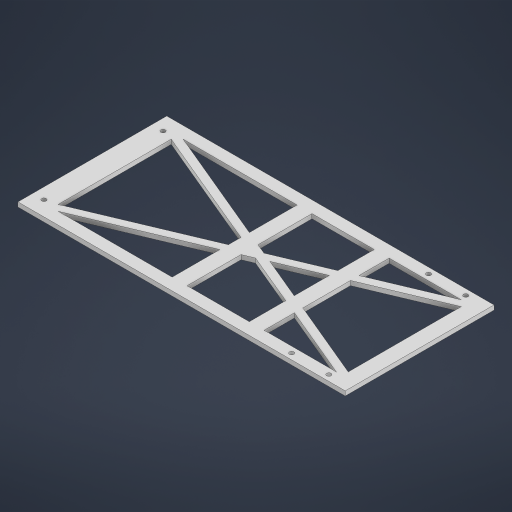
# Autodesk Inventor part: lf-esp
Saved by Autodesk Inventor 2023 (Build 270158000, 158)
## iProperties
Created: 2023-11-15
Part Number: lf-esp
Material: Ogólny
Document SubType Name: Modeling
Designer: mt150
Density: 1 g/cm^3
Appearance: Domyślna
Author: mt150
Autodesk Inventor part; units mm, degrees
ref_plane "YZ Plane" through (0, 0, 0) normal (1, 0, 0) x (0, 1, 0)
ref_plane "XZ Plane" through (0, 0, 0) normal (0, 1, 0) x (-1, 0, 0)
ref_plane "XY Plane" through (0, 0, 0) normal (0, 0, 1) x (1, 0, 0)
sketch "Szkic1" plane through (0, 0, 0) normal (0, 1, 0) x (-1, 0, 0)
  point P0 (0, 0)
sketch "Szkic2" plane through (0, 0, 0) normal (0, 1, 0) x (-1, 0, 0)
  line L0 (0, 0) -> (-15, 0)
  line L1 (-15, 0) -> (-15, 100)
  line L2 (-15, 100) -> (0, 100)
  line L3 (0, 100) -> (0, 0)
  line L4 (-7.5, 100) -> (-7.5, 90) construction
  line L5 (-7.5, 0) -> (-7.5, 10) construction
  circle A0 centre (-7.5, 90) radius 1.5
  circle A1 centre (-7.5, 10) radius 1.5
  line L6 (-15, 100) -> (-220, 100)
  line L7 (-220, 100) -> (-220, 92)
  line L8 (-220, 92) -> (-15, 92)
  line L9 (-15, 92) -> (-15, 100)
  line L10 (-15, 0) -> (-220, 0)
  line L11 (-220, 0) -> (-220, 8)
  line L12 (-220, 8) -> (-15, 8)
  line L13 (-15, 8) -> (-15, 0)
  line L14 (-15, 92) -> (-19, 92) construction
  line L15 (-15, 92) -> (-15, 88) construction
  line L16 (-220, 8) -> (-216, 8) construction
  line L17 (-220, 8) -> (-210, 8)
  line L18 (-210, 8) -> (-210, 92)
  line L19 (-210, 92) -> (-220, 92)
  line L20 (-220, 92) -> (-220, 8)
  line L21 (-210, 8) -> (-206, 8) construction
  line L22 (-210, 8) -> (-210, 12) construction
  line L23 (-15, 88) -> (-206, 8)
  line L24 (-19, 92) -> (-210, 12)
  line L25 (-15, 8) -> (-15, 12) construction
  line L26 (-15, 8) -> (-19, 8) construction
  line L27 (-210, 92) -> (-206, 92) construction
  line L28 (-210, 92) -> (-210, 88) construction
  line L29 (-210, 88) -> (-19, 8)
  line L30 (-15, 12) -> (-206, 92)
  line L31 (-220, 96) -> (-205, 96) construction
  line L32 (-220, 4) -> (-205, 4) construction
  circle A2 centre (-205, 96) radius 1.5
  circle A3 centre (-205, 4) radius 1.5
  line L33 (-205, 96) -> (-180, 96) construction
  line L34 (-205, 4) -> (-180, 4) construction
  circle A4 centre (-180, 96) radius 1.5
  circle A5 centre (-180, 4) radius 1.5
  line L35 (-220, 100) -> (-95, 100) construction
  line L36 (-95.6423, 92) -> (-105.6423, 92)
  line L37 (-105.6423, 92) -> (-105.6423, 8)
  line L38 (-105.6423, 8) -> (-95.6423, 8)
  line L39 (-95.6423, 8) -> (-95.6423, 92)
  line L40 (-220, 0) -> (-157.5, 0) construction
  line L41 (-157.5, 8) -> (-147.5, 8)
  line L42 (-147.5, 8) -> (-147.5, 92)
  line L43 (-147.5, 92) -> (-157.5, 92)
  line L44 (-157.5, 92) -> (-157.5, 8)
  point P0 (-105.725, 50)
  point P1 (-105.6423, 50.0346)
  point P2 (-105.6423, 49.9654)
  point P3 (-112.5, 52.8377)
  point P4 (-147.5, 67.4974)
  point P5 (-105.6423, 55.71)
  point P6 (-119.275, 50)
  point P7 (-147.5, 38.178)
  point P8 (-147.5, 61.822)
  point P9 (-112.5, 47.1623)
  point P10 (-105.6423, 44.29)
  point P11 (-147.5, 32.5026)
  point P12 (-157.5, 66.0105)
  point P13 (-157.5, 33.9895)
  point P14 (-157.5, 28.3141)
  point P15 (-157.5, 71.6859)
  point P16 (-95.6423, 59.8985)
  point P17 (-95.6423, 45.7769)
  point P18 (-95.6423, 54.2231)
  point P19 (-95.6423, 40.1015)
  dimension "d0" = 15
  dimension "d1" = 100
  dimension "d2" = 10
  dimension "d3" = 10
  dimension "d4" = 3
  dimension "d5" = 3
  dimension "d6" = 205
  dimension "d7" = 8
  dimension "d8" = 205
  dimension "d9" = 8
  dimension "d10" = 4
  dimension "d11" = 4
  dimension "d12" = 4
  dimension "d13" = 10
  dimension "d14" = 4
  dimension "d15" = 4
  dimension "d16" = 4
  dimension "d17" = 4
  dimension "d18" = 207.0773
  dimension "d19" = 15
  dimension "d20" = 15
  dimension "d21" = 3
  dimension "d22" = 3
  dimension "d23" = 25
  dimension "d24" = 3
  dimension "d25" = 3
  dimension "d26" = 125
  dimension "d27" = 10
  dimension "d28" = 10
  constraints: 90 end point, 16 point on line, 13 parallel, 10 horizontal, 6 centre point, 6 coincident, 6 perpendicular, 4 midpoint, 2 vertical
  measures "d0" distance of L1.end L2.end
  measures "d1" distance of L0.end L1.end
  measures "d2" distance of L4.start L4.end
  measures "d3" distance of L5.start L5.end
  measures "d4" diameter of A0
  measures "d5" diameter of A1
  measures "d6" distance of L8.end L7.end
  measures "d7" distance of L6.end L7.end
  measures "d8" distance of L11.end L12.end
  measures "d9" distance of L10.end L11.end
  measures "d10" distance of L8.end L14.end
  measures "d11" distance of L8.end L15.end
  measures "d12" distance of L11.end L16.end
  measures "d13" distance of L19.end L18.end
  measures "d14" distance of L17.end L21.end
  measures "d15" distance of L17.end L22.end
  measures "d16" distance of L12.end L25.end
  measures "d17" distance of L12.end L26.end
  measures "d18" distance of L25.end L27.end
  measures "d19" distance of L31.start L31.end
  measures "d20" distance of L32.start L32.end
  measures "d21" diameter of A2
  measures "d22" diameter of A3
  measures "d23" distance of L33.start L33.end
  measures "d24" diameter of A4
  measures "d25" diameter of A5
  measures "d26" distance of L6.end L35.end
  measures "d27" distance of L38.end L37.end
  measures "d28" distance of L43.end L42.end
extrude "Wyciągnięcie proste1" add sketch "Szkic2" along normal blind 3 contours L0 L1 L2 L3 | L10 L11 L12 L1 | L12 L29 L39 L30 L1 | L1 L8 L7 L6 | L20 L8 L18 L12 | L1 L23 L39 L24 L8 | L39 L29 L37 L30 | L30 L37 L23 L39 | L12 L37 L29 L39 | L18 L24 L44 L23 L12 | L23 L37 L24 L39 | L37 L29 L23 L30 | L30 L23 L37 | L8 L30 L44 L29 L18 | L39 L24 L37 L8 | L23 L30 L24 L37 | L23 L29 L24 L30 | L12 L44 L23 L42 | L23 L42 L24 L29 | L44 L24 L42 L23 | L44 L29 L42 L24 | L24 L29 L42 L30 | L44 L30 L42 L29 | L8 L42 L30 L44
